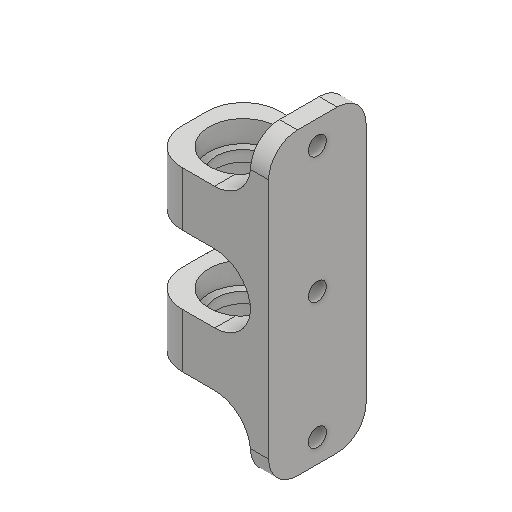
# Autodesk Inventor part: 3DP_ABS_Y_Axis_Pulley_Rod_Center_Bearing_Block
Saved by Autodesk Inventor 2026.1 (Build 301233000, 233)
## iProperties
Created: 2016-06-19
Part Number: 3DP_ABS_Y_Axis_Pulley_Rod_Center_Bearing_Block
Material: Ogólny
Document SubType Name: Modeling
Designer: Andrzej
Density: 1 g/cm^3
Appearance: Domyślna
Mass: 27.1938 g
Surface Area: 107.443 cm^2
Volume: 27.1938 cm^3
Author: Andrzej
Autodesk Inventor part; units mm, degrees
ref_plane "YZ Plane" through (0, 0, 0) normal (1, 0, 0) x (0, 1, 0)
ref_plane "XZ Plane" through (0, 0, 0) normal (0, 1, 0) x (-1, 0, 0)
ref_plane "XY Plane" through (0, 0, 0) normal (0, 0, 1) x (1, 0, 0)
sketch "Szkic1" plane through (0, 0, 0) normal (0, 0, 1) x (1, 0, 0)
  line L0 (-15.5705, 13.388) -> (18.4295, 13.388)
  line L1 (18.4295, 13.388) -> (18.4295, -13.612)
  line L2 (18.4295, -13.612) -> (-15.5705, -13.612)
  line L3 (-15.5705, -13.612) -> (-15.5705, 13.388)
  circle A0 centre (-2.0705, -0.112) radius 9.5
  point P0 (0, 0)
  dimension "d0" = 27
  dimension "d1" = 34
  dimension "d2" = 20.5
  dimension "d3" = 13.5
  dimension "d4" = 19
  constraints: 8 end point, 2 parallel, 1 centre point, 1 coincident, 1 horizontal, 1 perpendicular
  measures "d0" distance of L0.end L1.end
  measures "d1" distance of L1.end L2.end
  measures "d2" distance from line of L1 point (-2.071, -0.112)
  measures "d3" distance from line of point (-2.071, -0.112) L0
  measures "d4" diameter of A0
extrude "Wyciągnięcie proste1" add sketch "Szkic1" along normal blind 15 contours L0 L1 L2 L3 | A0
extrude "Wyciągnięcie proste2" cut sketch "Szkic1" along normal blind 6 contours A0
sketch "Szkic2" plane through (0, 0, 15) normal (0, 0, 1) x (1, 0, 0)
  circle A0 centre (-2.0705, -0.112) radius 9.5 projected
  line L0 (18.4295, 13.388) -> (-15.5705, 13.388) projected
  line L1 (-15.5705, 13.388) -> (-15.5705, -13.612) projected
  line L2 (-15.5705, -13.612) -> (18.4295, -13.612) projected
  line L3 (18.4295, -13.612) -> (18.4295, 13.388) projected
  point P0 (0, 0)
extrude "Wyciągnięcie proste3" cut sketch "Szkic2" against normal blind 6 contours A0
fillet "Zaokrąglenie1" radius 10 2 edges at (-15.5705, 13.388, 7.5) (-15.5705, -13.612, 7.5)
sketch "Szkic3" plane through (18.4295, -13.612, 0) normal (1, 0, 0) x (0, 0, -1)
  line L0 (0, 27) -> (0, 0) projected
  line L1 (0, 27) -> (-15, 27) projected
  line L2 (-15, 0) -> (-15, 27) projected
  line L3 (0, 0) -> (-15, 0) projected
  line L4 (-15, 27) -> (-34, 27)
  line L5 (-34, 27) -> (-34, 0)
  line L6 (-34, 0) -> (-15, 0)
  line L7 (0, 27) -> (17, 27)
  line L8 (17, 27) -> (17, 0)
  line L9 (17, 0) -> (0, 0)
  line L10 (-34, 27) -> (-49, 27)
  line L11 (-49, 27) -> (-49, 0)
  line L12 (-49, 0) -> (-34, 0)
  line L13 (-34, 0) -> (-34, 27)
  line L14 (-49, 27) -> (-66, 27)
  line L15 (-66, 27) -> (-66, 0)
  line L16 (-66, 0) -> (-49, 0)
  line L17 (-49, 0) -> (-49, 27)
  point P0 (0, 13.612)
  point P1 (-59.5, 13.5)
  point P2 (-24.5, 13.5)
  point P3 (10.5, 13.5)
  dimension "d26" = 13.5
  dimension "d21" = 19
  dimension "d22" = 17
  dimension "d25" = 27
  dimension "d41" = 15
  dimension "d42" = 15
  dimension "d43" = 27
  dimension "d44" = 17
  dimension "d45" = 27
  dimension "d50" = 13.5
  dimension "d51" = 6.5
  dimension "d58" = 9.5
  dimension "d59" = 6.5
  dimension "d60" = 13.5
  dimension "d61" = 13.5
  constraints: 28 end point, 5 perpendicular, 4 parallel, 3 horizontal, 1 point on line, 1 vertical
  measures "d21" distance of L1.end L4.end
  measures "d22" distance of L0.start L7.end
  measures "d25" distance of L4.end L5.end
  measures "d41" distance between parallel lines of L0 L2
  measures "d42" distance of L4.end L10.end
  measures "d43" distance of L10.end L11.end
  measures "d44" distance of L16.end L15.end
  measures "d45" distance of L14.end L15.end
  measures "d50" distance from line of L14 point (-59.5, 13.5)
  measures "d51" distance from line of point (-59.5, 13.5) L15
  measures "d58" distance from line of L13 point (-24.5, 13.5)
  measures "d59" distance from line of L8 point (10.5, 13.5)
  measures "d60" distance from line of L7 point (10.5, 13.5)
  measures "d61" distance from line of L4 point (-24.5, 13.5)
extrude "Wyciągnięcie proste4" add sketch "Szkic3" against normal blind 5 contours L7 L8 L9 L0 | L2 L6 L5 L4
extrude "Wyciągnięcie proste6" add sketch "Szkic3" against normal up to surface (34 mm away) contours L5 L12 L11 L10
extrude "Wyciągnięcie proste7" add sketch "Szkic3" against normal up to surface (5 mm away) contours L11 L16 L15 L14
hole "Otwór1" at (-2.0705, -0.112, 0) direction (0, 0, 1) diameter 15 end through all
fillet "Zaokrąglenie4" radius 10 2 edges at (-15.5705, 13.388, 41.5) (-15.5705, -13.612, 41.5)
sketch "Szkic5" plane through (13.4295, -13.612, 49) normal (0, 0, 1) x (1, 0, 0)
  circle A0 centre (-15.5, 13.5) radius 9.5 projected
  point P0 (-13.4295, 13.612)
extrude "Wyciągnięcie proste8" cut sketch "Szkic5" against normal blind 6
sketch "Szkic6" plane through (13.4295, -13.612, 34) normal (0, 0, -1) x (-1, 0, 0)
  circle A0 centre (15.5, 13.5) radius 9.5 projected
  arc A1 (19, 0) -> (29, 10) centre (19, 10) ccw projected
  line L0 (0, 0) -> (19, 0) projected
  line L1 (0, 0) -> (0, 27) projected
  line L2 (0, 27) -> (19, 27) projected
  arc A2 (29, 17) -> (19, 27) centre (19, 17) ccw projected
  line L3 (29, 17) -> (29, 10) projected
  point P0 (13.4295, 13.612)
extrude "Wyciągnięcie proste9" cut sketch "Szkic6" against normal blind 6 contours A0
fillet "Zaokrąglenie5" radius 10 4 edges at (13.4295, -0.112, 34) (13.4295, -0.112, 15) (13.4295, -0.112, 0) (13.4295, -0.112, 49)
hole "Otwór3" at (18.4295, -0.112, 59.5) at (18.4295, -0.112, 24.5) at (18.4295, -0.112, -10.5) direction (-1, 0, 0) diameter 5 end through all
sketch "Szkic7" plane through (13.4295, -13.612, 66) normal (-1, 0, 0) x (0, 0, 1)
  circle A0 centre (-6.5, 13.5) radius 5
  circle A1 centre (-41.5, 13.5) radius 5
  circle A2 centre (-76.5, 13.5) radius 5
  point P0 (-66, 13.612)
  dimension "d69" = 10
  dimension "d70" = 10
  dimension "d71" = 10
  constraints: 3 centre point, 3 coincident
  measures "d69" diameter of A0
  measures "d70" diameter of A1
  measures "d71" diameter of A2
extrude "Wyciągnięcie proste10" cut sketch "Szkic7" along normal blind 6
fillet "Zaokrąglenie6" radius 8 4 edges at (15.9295, 13.388, 66) (15.9295, -13.612, 66) (15.9295, 13.388, -17) (15.9295, -13.612, -17)
equation "\"d3\" = 0.5 * d0"
equation "\"d26\" = 0.5 * d25"
equation "\"d42\" = d41"
equation "\"d50\" = d26"
equation "\"d58\" = 0.5 * d21"
equation "\"d59\" = d51"
equation "\"d60\" = 0.5 * d43"
equation "\"d61\" = d60"
